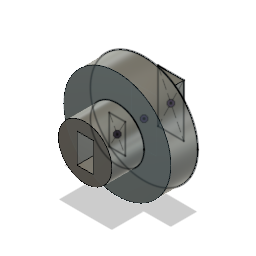
Gear to Motor Mount (Autodesk Fusion 360 design; units mm, degrees)
Autodesk Fusion 360 part; units mm, degrees
sketch "Sketch1" plane through (0, 0, 0) normal (0, 0, 1) x (1, 0, 0)
  line L0 (2.4, 4.9) -> (-2.4, 4.9)
  line L1 (-2.4, 4.9) -> (-2.4, -4.9)
  line L2 (-2.4, -4.9) -> (2.4, -4.9)
  line L3 (2.4, -4.9) -> (2.4, 4.9)
  line L4 (2.4, 4.9) -> (-2.4, -4.9) construction
  line L5 (-2.4, 4.9) -> (2.4, -4.9) construction
  dimension "d1" = 4.8
  dimension "d2" = 9.8
  constraint perpendicular L0 L1
  constraint parallel L0 L2
  constraint parallel L1 L3
  constraint horizontal L0
  constraint coincident L4 origin
  constraint coincident L5 origin
  measures "d1" distance of L1.end L2.end
  measures "d2" distance of L0.end L1.end
extrude "Extrude1" add sketch "Sketch1" along normal blind 5
sketch "Sketch2" plane through (0, 0, 5) normal (0, 0, 1) x (1, 0, 0)
  line L0 (2.4, -4.9) -> (2.4, 4.9)
  line L1 (2.4, 4.9) -> (-2.4, 4.9)
  line L2 (-2.4, 4.9) -> (-2.4, -4.9)
  line L3 (-2.4, -4.9) -> (2.4, -4.9)
  circle A0 centre (0, 0) radius 10
  dimension "d5" = 20
  constraint coincident A0.centre origin
  measures "d5" diameter of A0
extrude "Extrude2" add sketch "Sketch2" along normal blind 5 contours L0 L1 L2 L3 | A0
sketch "Sketch3" plane through (0, 0, 10) normal (0, 0, 1) x (1, 0, 0)
  circle A0 centre (0, 0) radius 10
  line L0 (-1.5, 2.75) -> (1.5, 2.75)
  line L1 (1.5, 2.75) -> (1.5, -2.75)
  line L2 (1.5, -2.75) -> (-1.5, -2.75)
  line L3 (-1.5, -2.75) -> (-1.5, 2.75)
  line L4 (-1.5, 2.75) -> (1.5, -2.75) construction
  line L5 (1.5, 2.75) -> (-1.5, -2.75) construction
  circle A1 centre (0, 0) radius 5
  dimension "d8" = 5.5
  dimension "d9" = 3
  dimension "d10" = 10
  constraint perpendicular L0 L1
  constraint parallel L0 L2
  constraint parallel L1 L3
  constraint horizontal L0
  constraint coincident L4 A0.centre
  constraint coincident L5 A0.centre
  constraint coincident A0.centre A1.centre
  measures "d8" distance of L0.end L1.end
  measures "d9" distance of L1.end L2.end
  measures "d10" diameter of A1
extrude "Extrude3" add sketch "Sketch3" along normal blind 6 contours A1
extrude "Extrude4" cut sketch "Sketch3" against normal blind 3 contours L0 L1 L2 L3
